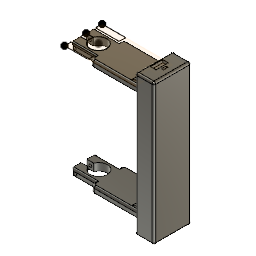
Trekking_Pole_Adapter_shanjingxuan (Autodesk Fusion 360 design; units mm, degrees)
Autodesk Fusion 360 part; units mm, degrees
sketch "Sketch1" plane through (0, 0, 0) normal (0, 0, 1) x (1, 0, 0) in component "Case"
  line L0 (-10, 20) -> (10, 20)
  line L1 (10, 20) -> (10, -20)
  line L2 (10, -20) -> (-10, -20)
  line L3 (-10, -20) -> (-10, 20)
  dimension "d1" = 20
  dimension "d2" = 40
  dimension "d3" = 20
  dimension "d4" = 10
  constraint horizontal L0
  constraint vertical L1
  constraint horizontal L2
  constraint vertical L3
  measures "d1" distance of L0.start L0.end
  measures "d2" distance of L0.start L2.end
  measures "d3" vertical distance of origin L0.start
  measures "d4" horizontal distance of origin L0.start
extrude "Extrude1" add sketch "Sketch1" along normal blind 150 makes body 1 in component "Case"
shell "Shell1" thickness 3 removed faces 1 at (-10, -6.6667, 50) on bodies 1 in component "Case"
sketch "Sketch2" plane through (0, 0, 150) normal (0, 0, 1) x (-1, 0, 0) in component "Case"
  line L0 (10, 20) -> (-10, 20)
  line L1 (-10, 20) -> (-10, -20)
  line L2 (-10, -20) -> (10, -20)
  line L3 (10, -20) -> (10, 20)
  line L4 (7, -6.5) -> (1.2, -6.5)
  line L5 (1.2, -6.5) -> (1.2, 6.5)
  line L6 (1.2, 6.5) -> (7, 6.5)
  line L7 (7, 6.5) -> (7, -6.5)
  line L8 (-0.8, -2.5) -> (-2.8, -2.5)
  line L9 (-2.8, -2.5) -> (-2.8, 2.5)
  line L10 (-2.8, 2.5) -> (-0.8, 2.5)
  line L11 (-0.8, 2.5) -> (-0.8, -2.5)
  dimension "d8" = 5.8
  dimension "d9" = 13
  dimension "d10" = 3
  dimension "d11" = 13.5
  dimension "d12" = 2
  dimension "d13" = 5
  dimension "d14" = 17.5
  dimension "d15" = 2
  constraint horizontal L4
  constraint vertical L5
  constraint horizontal L6
  constraint vertical L7
  constraint horizontal L8
  constraint vertical L9
  constraint horizontal L10
  constraint vertical L11
  measures "d8" distance of L4.start L4.end
  measures "d9" distance of L4.start L6.end
  measures "d10" horizontal distance of L0.start L6.end
  measures "d11" vertical distance of L0.start L6.end
  measures "d12" distance of L8.start L8.end
  measures "d13" distance of L8.start L10.end
  measures "d14" vertical distance of L0.end L9.end
  measures "d15" horizontal distance of L5.end L10.end
extrude "Extrude2" cut sketch "Sketch2" against normal blind 4 contours L4 L5 L6 L7 | L8 L9 L10 L11 bodies 1 in component "Case"
fillet "Fillet1" radius 2 8 edges at (0, -20, 150) (10, -20, 75) (0, -20, 0) (10, 0, 0) (0, 20, 0) (10, 20, 75) (0, 20, 150) (10, 0, 150) on bodies 1 in component "Case"
fillet "Fillet1" radius 2 4 edges at (-10, 20, 75) (-10, 0, 150) (-10, -20, 75) (-10, 0, 0) on bodies 1 in component "Case"
sketch "Sketch5" plane through (0, 0, 147) normal (0, 0, -1) x (1, 0, 0) in component "Case"
  line L0 (-1.2, 6.5) -> (-1.2, -6.5)
  line L1 (-1.2, -6.5) -> (-7, -6.5)
  line L2 (-7, -6.5) -> (-7, 6.5)
  line L3 (-7, 6.5) -> (-1.2, 6.5)
  line L4 (2.8, 2.5) -> (2.8, -2.5)
  line L5 (2.8, -2.5) -> (0.8, -2.5)
  line L6 (0.8, -2.5) -> (0.8, 2.5)
  line L7 (0.8, 2.5) -> (2.8, 2.5)
  line L8 (7, 17) -> (-10, 17)
  line L9 (-10, 17) -> (-10, -17)
  line L10 (-10, -17) -> (7, -17)
  line L11 (7, -17) -> (7, 17)
ref_plane "WorkPlane1" through (-7, 0, 75) normal (-1, 0, 0) x (0, -1, 0) in component "Case"
sketch "Sketch6" plane through (-7, 0, 75) normal (-1, 0, 0) x (0, 1, 0) in component "Case"
  line L0 (-11, 66) -> (-17, 66)
  line L1 (-17, 66) -> (-17, 72)
  line L2 (-17, 72) -> (-11, 72)
  line L3 (-11, 72) -> (-11, 66)
  line L4 (17, 72) -> (11, 72)
  line L5 (11, 72) -> (11, 66)
  line L6 (11, 66) -> (17, 66)
  line L7 (17, 66) -> (17, 72)
  line L8 (-11, -72) -> (-17, -72)
  line L9 (-17, -72) -> (-17, -66)
  line L10 (-17, -66) -> (-11, -66)
  line L11 (-11, -66) -> (-11, -72)
  line L12 (18, -75) -> (-18, -75)
  line L13 (17, -72) -> (11, -72)
  line L14 (11, -72) -> (11, -66)
  line L15 (11, -66) -> (17, -66)
  line L16 (17, -66) -> (17, -72)
  line L17 (20, 73) -> (20, -73)
  point P0 (-17, 72)
  point P1 (-18, 75)
  point P2 (-20, 73)
  point P3 (20, 73)
  point P4 (18, 75)
  point P5 (-20, -73)
  dimension "d48" = 6
  dimension "d49" = 6
  dimension "d51" = 3
  dimension "d52" = 3
  dimension "d53" = 6
  dimension "d54" = 6
  dimension "d55" = 3
  dimension "d56" = 3
  dimension "d57" = 6
  dimension "d58" = 6
  dimension "d59" = 3
  dimension "d60" = 3
  dimension "d61" = 6
  dimension "d62" = 6
  dimension "d63" = 3
  dimension "d64" = 3
  constraint horizontal L0
  constraint vertical L1
  constraint horizontal L2
  constraint vertical L3
  constraint horizontal L4
  constraint vertical L5
  constraint horizontal L6
  constraint vertical L7
  constraint horizontal L8
  constraint vertical L9
  constraint horizontal L10
  constraint vertical L11
  constraint horizontal L13
  constraint vertical L14
  constraint horizontal L15
  constraint vertical L16
  measures "d48" distance of L0.start L0.end
  measures "d49" distance of L0.start L2.end
  measures "d51" vertical distance of P0 P1
  measures "d52" horizontal distance of P0 P2
  measures "d53" distance of L4.start L6.end
  measures "d54" distance of L4.start L4.end
  measures "d55" horizontal distance of L4.start P3
  measures "d56" vertical distance of L4.start P4
  measures "d57" distance of L8.start L8.end
  measures "d58" distance of L8.start L10.end
  measures "d59" horizontal distance of L8.end P5
  measures "d60" distance of L8.end L12
  measures "d61" distance of L13.start L13.end
  measures "d62" distance of L13.start L15.end
  measures "d63" vertical distance of L12.start L13.start
  measures "d64" distance of L13.start L17
extrude "Extrude5" add sketch "Sketch6" against normal blind 6 bodies 1 in component "Case"
draft "Draft1" angle 45 neutral plane through (-7, -17, 141) pull (0, 0, -1) 1 faces at (-1, -13, 145) on bodies 1 in component "Case"
draft "Draft2" angle 45 neutral plane through (-7, 11, 141) pull (0, 0, -1) 1 faces at (-1, 13, 143) on bodies 1 in component "Case"
draft "Draft3" angle 45 neutral plane through (-7, 11, 9) pull (0, 0, 1) 1 faces at (-1, 13, 7) on bodies 1 in component "Case"
draft "Draft4" angle 45 neutral plane through (-7, -11, 9) pull (0, 0, 1) 1 faces at (-1, -13, 7) on bodies 1 in component "Case"
hole "Hole5" at (-10, -14, 144) direction (1, 0, 0) diameter 2 depth 6 tip angle 118 bodies 1 in component "Case"
hole "Hole6" at (-7, 14, 144) direction (1, 0, 0) diameter 2 depth 6 tip angle 118 bodies 1 in component "Case"
hole "Hole7" at (-7, -14, 6) direction (1, 0, 0) diameter 2 depth 6 tip angle 118 bodies 1 in component "Case"
hole "Hole8" at (-7, 14, 6) direction (1, 0, 0) diameter 2 depth 6 tip angle 118 bodies 1 in component "Case"
sketch "Sketch1 (2)" plane through (-7, 0, 0) normal (-1, 0, 0) x (0, -1, 0) in component "Side"
  circle A0 centre (14, 6) radius 1
  line L0 (11, 3) -> (17, 3)
  line L1 (17, 3) -> (17, 9)
  line L2 (17, 9) -> (11, 9)
  line L3 (11, 9) -> (11, 3)
  circle A1 centre (-14, 6) radius 1
  line L4 (-17, 9) -> (-17, 3)
  line L5 (-17, 3) -> (-11, 3)
  line L6 (-11, 3) -> (-11, 9)
  line L7 (-11, 9) -> (-17, 9)
  circle A2 centre (14, 144) radius 1
  line L8 (11, 141) -> (17, 141)
  line L9 (17, 141) -> (17, 147)
  line L10 (17, 147) -> (11, 147)
  line L11 (11, 147) -> (11, 141)
  circle A3 centre (-14, 144) radius 1
  line L12 (-17, 141) -> (-11, 141)
  line L13 (-11, 141) -> (-11, 147)
  line L14 (-11, 147) -> (-17, 147)
  line L15 (-17, 147) -> (-17, 141)
  line L16 (-17, 3) -> (17, 3)
  line L17 (17, 3) -> (17, 147)
  line L18 (17, 147) -> (-17, 147)
  line L19 (-17, 147) -> (-17, 3)
extrude "Extrude1'" add sketch "Sketch1 (2)" along normal blind 3 separate body makes body 2 in component "Side"
sketch "Sketch2 (2)" plane through (-10, 0, 0) normal (-1, 0, 0) x (0, -1, 0) in component "Side"
  circle A0 centre (14, 144) radius 1
  circle A1 centre (-14, 144) radius 1
  circle A2 centre (14, 6) radius 1
  circle A3 centre (-14, 6) radius 1
  line L0 (-17, 147) -> (-17, 3)
  line L1 (-17, 3) -> (17, 3)
  line L2 (17, 3) -> (17, 147)
  line L3 (17, 147) -> (-17, 147)
  line L4 (-15, 137) -> (15, 137)
  line L5 (15, 137) -> (15, 129)
  line L6 (15, 129) -> (-15, 129)
  line L7 (-15, 129) -> (-15, 137)
  line L8 (-15, 21) -> (15, 21)
  line L9 (15, 21) -> (15, 13)
  line L10 (15, 13) -> (-15, 13)
  line L11 (-15, 13) -> (-15, 21)
  point P0 (-17, 147)
  dimension "d91" = 30
  dimension "d92" = 8
  dimension "d93" = 10
  dimension "d94" = 2
  dimension "d95" = 30
  dimension "d96" = 8
  dimension "d97" = 10
  dimension "d98" = 2
  dimension "d109" = 124
  constraint horizontal L4
  constraint vertical L5
  constraint horizontal L6
  constraint vertical L7
  constraint horizontal L8
  constraint vertical L9
  constraint horizontal L10
  constraint vertical L11
  measures "d91" distance of L4.start L4.end
  measures "d92" distance of L4.start L6.end
  measures "d93" vertical distance of P0 L4.start
  measures "d94" horizontal distance of L4.start P0
  measures "d95" distance of L8.start L8.end
  measures "d96" distance of L8.start L10.end
  measures "d97" vertical distance of L0.end L10.end
  measures "d98" horizontal distance of L0.end L10.end
  measures "d109" distance of L4.start L10.end
extrude "Extrude2'" add sketch "Sketch2 (2)" along normal blind 8 contours L4 L5 L6 L7 | L8 L9 L10 L11 bodies 2 in component "Side"
draft "Draft1'" angle -30 neutral plane through (-18, 0, 0) pull (-1, 0, 0) 1 faces at (-12.6667, -15, 134.3333) on bodies 2 in component "Side"
draft "Draft2'" angle -30 neutral plane through (-18, 0, 0) pull (-1, 0, 0) 1 faces at (-12.6667, 15, 131.6667) on bodies 2 in component "Side"
draft "Draft3'" angle -30 neutral plane through (-18, 0, 0) pull (-1, 0, 0) 1 faces at (-12.6667, 15, 15.6667) on bodies 2 in component "Side"
draft "Draft4'" angle -30 neutral plane through (-18, 0, 0) pull (-1, 0, 0) 1 faces at (-12.6667, -15, 18.3333) on bodies 2 in component "Side"
sketch "Sketch1 (3)" plane through (0, 0, 137) normal (0, 0, 1) x (-1, 0, 0) in component "Holder"
  line L0 (10, 10.3812) -> (10, -10.3812)
  line L1 (10, -10.3812) -> (18, -15)
  line L2 (18, -15) -> (18, 15)
  line L3 (18, 15) -> (10, 10.3812)
  line L4 (10, -20) -> (85, -20)
  line L5 (85, -20) -> (85, 20)
  line L6 (85, 20) -> (10, 20)
  line L7 (10, 20) -> (10, -20)
  line L8 (8, 20) -> (-8, 20)
  dimension "d110" = 75
  dimension "d111" = 40
  dimension "d140" = 40
  constraint horizontal L4
  constraint vertical L5
  constraint horizontal L6
  constraint vertical L7
  measures "d110" distance of L4.start L4.end
  measures "d111" distance of L4.start L6.end
  measures "d140" distance of L4.start L8
extrude "Extrude1''" add sketch "Sketch1 (3)" against normal blind 8 separate body contours L1 L2 L3 L4 L5 L6 L7 makes body 3 in component "Holder"
move_face "OffsetFaces1" offset -0.2 1 faces at (-12.6667, 11.9208, 134.3333) on bodies 3 in component "Holder"
move_face "OffsetFaces2" offset -0.2 1 faces at (-15.3333, -13.4604, 134.3333) on bodies 3 in component "Holder"
move_face "OffsetFaces3" offset -0.2 1 faces at (-18, 5.077, 134.3333) on bodies 3 in component "Holder"
sketch "Sketch2 (3)" plane through (0, 0, 137) normal (0, 0, 1) x (-1, 0, 0) in component "Holder"
  line L0 (10, -10.6121) -> (10, -20)
  line L1 (10, -20) -> (85, -20)
  line L2 (85, -20) -> (85, 20)
  line L3 (85, 20) -> (10, 20)
  line L4 (10, 20) -> (10, 10.6121)
  line L5 (10, 10.6121) -> (18.2, 15.3464)
  line L6 (18.2, 15.3464) -> (18.2, -15.3464)
  line L7 (18.2, -15.3464) -> (10, -10.6121)
  circle A0 centre (69, 0) radius 9
  line L8 (85, -20) -> (60, -20)
  line L9 (60, -20) -> (60, -13)
  line L10 (60, -13) -> (85, -13)
  line L11 (85, -13) -> (85, -20)
  line L12 (85, 20) -> (60, 20)
  line L13 (60, 20) -> (60, 13)
  line L14 (60, 13) -> (85, 13)
  line L15 (85, 13) -> (85, 20)
  line L16 (85, -3) -> (77.5, -3)
  line L17 (77.5, -3) -> (77.5, 3)
  line L18 (77.5, 3) -> (85, 3)
  line L19 (85, 3) -> (85, -3)
  dimension "d118" = 18
  dimension "d119" = 16
  dimension "d120" = 20
  dimension "d121" = 59
  dimension "d124" = 25
  dimension "d125" = 7
  dimension "d126" = 7
  dimension "d127" = 25
  dimension "d128" = 7.5
  dimension "d129" = 6
  dimension "d130" = 17
  constraint horizontal L8
  constraint vertical L9
  constraint horizontal L10
  constraint vertical L11
  constraint coincident L1.end L2.start
  constraint horizontal L12
  constraint vertical L13
  constraint horizontal L14
  constraint vertical L15
  constraint coincident L2.end L3.start
  constraint horizontal L16
  constraint vertical L17
  constraint horizontal L18
  constraint vertical L19
  constraint coincident L2 L16.start
  measures "d118" diameter of A0
  measures "d119" horizontal distance of L1.end A0.centre
  measures "d120" vertical distance of L1.end A0.centre
  measures "d121" horizontal distance of L0.end A0.centre
  measures "d124" distance of L1.end L8.end
  measures "d125" distance of L1.end L10.end
  measures "d126" distance of L2.end L14.end
  measures "d127" distance of L2.end L12.end
  measures "d128" distance of L16.start L16.end
  measures "d129" distance of L16.start L18.end
  measures "d130" distance of L1.end L16.start
extrude "Extrude3" cut sketch "Sketch2 (3)" against normal blind 10 contours L1 L2 L8 L9 L10 L11 | L2 A0 L16 L17 L18 L19 | L2 L3 L12 L13 L14 L15 | A0 L17 picked at (70.7248, 1.7533) bodies 3 in component "Holder"
extrude "Extrude2''" cut sketch "Sketch2 (3)" against normal blind 10 contours A0 L17 | A0 L17 bodies 3 in component "Holder"
sketch "Sketch3" plane through (0, -13, 0) normal (0, -1, 0) x (1, 0, 0) in component "Holder"
  line L0 (-85, 129) -> (-60, 129)
  line L1 (-60, 129) -> (-60, 137)
  line L2 (-60, 137) -> (-85, 137)
  line L3 (-85, 137) -> (-85, 129)
  circle A0 centre (-81, 133) radius 1.5
  point P0 (-85, 137)
  dimension "d133" = 3
  dimension "d134" = 4
  dimension "d135" = 4
  measures "d133" diameter of A0
  measures "d134" horizontal distance of P0 A0.centre
  measures "d135" vertical distance of A0.centre P0
extrude "Extrude4" cut sketch "Sketch3" against normal blind 30 contours A0 bodies 3 in component "Holder"
move_face "OffsetFaces4" offset -2 1 faces at (-43.3333, -20, 134.3333) on bodies 3 in component "Holder"
move_face "OffsetFaces5" offset -2 1 faces at (-26.6667, 20, 134.3333) on bodies 3 in component "Holder"
fillet "Fillet1'" radius 4 2 edges at (-60, 18, 133) (-60, -18, 133) on bodies 3 in component "Holder"
fillet "Fillet1'" radius 2 14 edges at (-72.5, 13, 137) (-35, 18, 137) (-60, 15.5, 137) (-35, -18, 137) (-60, -15.5, 137) (-72.5, -13, 137) (-85, 13, 133) (-85, -13, 133) (-72.5, -13, 129) (-60, -15.5, 129) (-35, -18, 129) (-72.5, 13, 129) (-35, 18, 129) (-60, 15.5, 129) on bodies 3 in component "Holder"
copy_body "CopyPasteBodies1" bodies 3 makes body 4 in component "Holder"
move_body "Move1" bodies 4 to x (1, 0, 0) y (0, 1, 0) z (0, 0, 1) at (0.2, 0.3464, -116) in component "Holder"
component "Holder" placed x (1, 0, 0) y (0, 1, 0) z (0, 0, 1) at (0, 0, 0)
component "Side" placed x (1, 0, 0) y (0, 1, 0) z (0, 0, 1) at (0, 0, 0)
component "Case" placed x (1, 0, 0) y (0, 1, 0) z (0, 0, 1) at (0, 0, 0)
